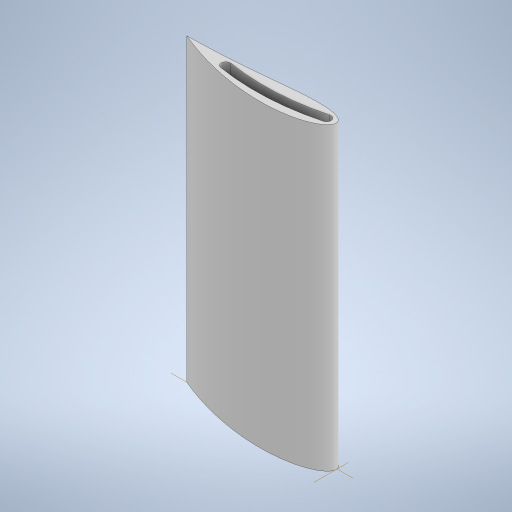
# Autodesk Inventor part: 5518
Saved by Autodesk Inventor 2023 (Build 270158000, 158)
## iProperties
Created: 2023-03-15
Part Number: 5518
Material: 一般
Document SubType Name: Modeling
Designer: USER
Density: 1 g/cm^3
Appearance: 預設
Author: USER
Autodesk Inventor part; units mm, degrees
ref_plane "YZ Plane" through (0, 0, 0) normal (1, 0, 0) x (0, 1, 0)
ref_plane "XZ Plane" through (0, 0, 0) normal (0, 1, 0) x (-1, 0, 0)
ref_plane "XY Plane" through (0, 0, 0) normal (0, 0, 1) x (1, 0, 0)
sketch "草圖2" plane through (0, 0, 0) normal (0, 1, 0) x (-1, 0, 0)
  spline S0 degree 5 poles (50, 0) (50.001, 0.0051) (49.9528, 0.0248) (49.7193, 0.0935) (49.7129, 0.1657) (49.0646, 0.3605) (48.7927, 0.541) (47.9768, 0.8251) (47.2986, 1.1244) (46.3079, 1.4873) (45.2886, 1.8729) (44.0856, 2.2932) (42.7927, 2.7296) (41.3704, 3.1801) (39.8497, 3.6332) (38.2275, 4.0826) (36.5184, 4.5196) (34.7298, 4.9366) (32.8733, 5.3263) (30.9599, 5.6817) (29.0015, 5.9961) (27.0109, 6.2637) (25.0008, 6.4789) (22.985, 6.6373) (20.977, 6.7348) (18.9909, 6.769) (17.0407, 6.7378) (15.1405, 6.6409) (13.3039, 6.4789) (11.5442, 6.2535) (9.8739, 5.9683) (8.3052, 5.6276) (6.8485, 5.2368) (5.5137, 4.8026) (4.309, 4.3322) (3.2414, 3.8328) (2.3161, 3.312) (1.5364, 2.7762) (0.9047, 2.2301) (0.4224, 1.6772) (0.0961, 1.1163) (-0.0649, 0.5529) (-0.0423, -0.0079) (0.1523, -0.5334) (0.5119, -0.9918) (1.0158, -1.3889) (1.6519, -1.7264) (2.4138, -2.0115) (3.2977, -2.2458) (4.3, -2.4315) (5.4156, -2.569) (6.6384, -2.6596) (7.9619, -2.7047) (9.3786, -2.7068) (10.8812, -2.6684) (12.4619, -2.5937) (14.1126, -2.4866) (15.825, -2.3525) (17.5907, -2.1963) (19.4008, -2.0239) (21.2462, -1.8406) (23.1174, -1.6519) (25.0045, -1.463) (26.8972, -1.2782) (28.7851, -1.1015) (30.6572, -0.9361) (32.5024, -0.7842) (34.3095, -0.6472) (36.0673, -0.5263) (37.7638, -0.4212) (39.3902, -0.332) (40.9302, -0.2565) (42.3843, -0.1961) (43.7202, -0.1437) (44.9715, -0.1094) (46.0467, -0.0689) (47.0887, -0.063) (47.8246, -0.0158) (48.6807, -0.0488) (49.0006, 0.0219) (49.6713, -0.0438) (49.7054, 0.0216) (49.9469, -0.0047) (49.999, -0.0051) (50, 0) knots 0 0 0 0 0 0 0.005562 0.010419 0.017175 0.02538 0.034731 0.045061 0.056244 0.068183 0.080795 0.094007 0.107751 0.121966 0.136593 0.151578 0.166867 0.182408 0.19815 0.214043 0.230037 0.246082 0.262129 0.27813 0.294034 0.309792 0.325355 0.340673 0.355696 0.370375 0.38466 0.398501 0.411849 0.424654 0.43687 0.448453 0.459371 0.469613 0.479205 0.488239 0.496858 0.505244 0.513623 0.522219 0.531206 0.540716 0.550832 0.561575 0.57293 0.584866 0.597341 0.61031 0.623731 0.637558 0.651748 0.666258 0.681046 0.696071 0.711288 0.726658 0.742136 0.757679 0.773244 0.788785 0.804257 0.819613 0.834805 0.849782 0.864492 0.878883 0.892897 0.906474 0.91955 0.932056 0.943914 0.955038 0.965326 0.974651 0.982839 0.989587 0.99444 1 1 1 1 1 1
  point P0 (49.7052, 0.1268)
  point P1 (49.3378, 0.2828)
  point P2 (48.8255, 0.4967)
  point P3 (48.1705, 0.7643)
  point P4 (47.3758, 1.0802)
  point P5 (46.4449, 1.4382)
  point P6 (45.382, 1.8315)
  point P7 (44.1923, 2.2525)
  point P8 (42.8818, 2.6935)
  point P9 (41.4571, 3.1465)
  point P10 (39.9258, 3.6031)
  point P11 (38.2963, 4.0553)
  point P12 (36.5777, 4.4952)
  point P13 (34.7799, 4.9149)
  point P14 (32.9136, 5.3069)
  point P15 (30.9903, 5.6643)
  point P16 (29.0217, 5.9802)
  point P17 (27.0206, 6.2489)
  point P18 (25, 6.4646)
  point P19 (22.9736, 6.6229)
  point P20 (20.9552, 6.7199)
  point P21 (18.959, 6.7527)
  point P22 (16.9991, 6.7195)
  point P23 (15.0896, 6.6199)
  point P24 (13.2444, 6.4545)
  point P25 (11.477, 6.2251)
  point P26 (9.8, 5.9351)
  point P27 (8.2256, 5.5888)
  point P28 (6.7649, 5.192)
  point P29 (5.4277, 4.7509)
  point P30 (4.2229, 4.273)
  point P31 (3.1582, 3.7659)
  point P32 (2.2397, 3.2374)
  point P33 (1.4727, 2.6951)
  point P34 (0.8607, 2.1465)
  point P35 (0.4065, 1.5979)
  point P36 (0.1115, 1.0548)
  point P37 (-0.0238, 0.5212)
  point P38 (0, 0)
  point P39 (0.1779, -0.4904)
  point P40 (0.5041, -0.9324)
  point P41 (0.975, -1.3254)
  point P42 (1.5865, -1.669)
  point P43 (2.3333, -1.9629)
  point P44 (3.2099, -2.2069)
  point P45 (4.2098, -2.4009)
  point P46 (5.3262, -2.5456)
  point P47 (6.552, -2.6421)
  point P48 (7.8798, -2.692)
  point P49 (9.3019, -2.6978)
  point P50 (10.8107, -2.6625)
  point P51 (12.3982, -2.5901)
  point P52 (14.0561, -2.485)
  point P53 (15.7763, -2.3521)
  point P54 (17.5501, -2.197)
  point P55 (19.3688, -2.0252)
  point P56 (21.2231, -1.8422)
  point P57 (23.1034, -1.6536)
  point P58 (25, -1.4646)
  point P59 (26.9024, -1.2796)
  point P60 (28.8001, -1.1026)
  point P61 (30.6821, -0.9368)
  point P62 (32.5372, -0.7844)
  point P63 (34.3543, -0.6471)
  point P64 (36.1218, -0.5257)
  point P65 (37.8286, -0.4204)
  point P66 (39.4634, -0.3306)
  point P67 (41.0153, -0.2554)
  point P68 (42.4735, -0.1935)
  point P69 (43.828, -0.1436)
  point P70 (45.0688, -0.104)
  point P71 (46.1872, -0.0732)
  point P72 (47.1745, -0.0497)
  point P73 (48.0234, -0.0321)
  point P74 (48.7274, -0.0192)
  point P75 (49.2807, -0.0103)
  point P76 (49.6793, -0.0044)
  point P77 (49.9197, -0.0011)
  constraints: 80 other
extrude "擠出1" add sketch "草圖2" along normal blind 100
sketch "草圖3" plane through (0, 100, 0) normal (0, 1, 0) x (1, 0, 0)
  arc A0 (-35, -2.0703) -> (-3, -0.4713) centre (-22.7332, 73.4398) ccw construction
  arc A1 (-35.2405, -3.5509) -> (-2.6131, -1.9205) centre (-22.7332, 73.4398) ccw
  arc A2 (-34.7595, -0.5897) -> (-3.3869, 0.978) centre (-22.7332, 73.4398) ccw
  arc A3 (-34.7595, -0.5897) -> (-35.2405, -3.5509) centre (-35, -2.0703) ccw
  arc A4 (-2.6131, -1.9205) -> (-3.3869, 0.978) centre (-3, -0.4713) ccw
  line L0 (0, 89.4747) -> (0, -22.8096) projected
  dimension "d3" = 1.5
  dimension "d5" = 3
  dimension "d6" = 32
  constraints: 10 point on circle, 5 centre point, 4 tangent
  measures "d3" radius of A4
  measures "d5" distance from line of L0 A0.end
  measures "d6" horizontal distance of A0.end A0.start
extrude "擠出2" cut sketch "草圖3" against normal through all
